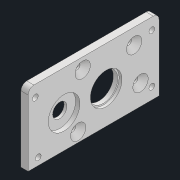
# Autodesk Inventor part: One Motor Plate
Saved by Autodesk Inventor 2022 (Build 260153000, 153)
## iProperties
Created: 2022-09-09
Part Number: One Motor Plate
Material: Generic
Document SubType Name: Modeling
Designer: robpl
Density: 1 g/cm^3
Appearance: Default
Author: robpl
Autodesk Inventor part; units mm, degrees
ref_plane "YZ Plane" through (0, 0, 0) normal (1, 0, 0) x (0, 1, 0)
ref_plane "XZ Plane" through (0, 0, 0) normal (0, 1, 0) x (-1, 0, 0)
ref_plane "XY Plane" through (0, 0, 0) normal (0, 0, 1) x (1, 0, 0)
sketch "Sketch1" plane through (0, 0, 0) normal (1, 0, 0) x (0, 1, 0)
  line L0 (0, 0) -> (50, 0)
  line L1 (50, 0) -> (50, -91)
  line L2 (50, -91) -> (0, -91)
  line L3 (0, -91) -> (0, 0)
  dimension "d0" = 50
  dimension "d1" = 91
  constraints: 8 end point, 2 parallel, 1 horizontal, 1 perpendicular
  measures "d0" distance of L1.end L2.end
  measures "d1" distance of L0.end L1.end
extrude "Extrusion1" add sketch "Sketch1" along normal blind 5
sketch "Sketch2" plane through (5, 0, 0) normal (1, 0, 0) x (0, 0, -1)
  line L0 (0, 0) -> (91, 0) projected
  line L1 (0, 50) -> (0, 0) projected
  point P0 (25, 22.8)
  dimension "d4" = 22.8
  dimension "d5" = 25
  measures "d4" distance from line of point (25, 22.8) L0
  measures "d5" distance from line of L1 point (25, 22.8)
hole "Hole1" at (5, 22.8, -25) direction (-1, 0, 0) diameter 10 end through all counterbore diameter 22 counterbore depth 3
sketch "Sketch3" plane through (5, 0, 0) normal (1, 0, 0) x (0, 0, -1)
  circle A0 centre (25, 22.8) radius 11 projected
  line L0 (91, 0) -> (91, 50) projected
  line L1 (91, 50) -> (0, 50) projected
  line L2 (0, 50) -> (0, 0) projected
  line L3 (0, 0) -> (91, 0) projected
  circle A1 centre (25, 22.8) radius 5 projected
  line L4 (25, 22.8) -> (54.26, 22.8)
  dimension "d13" = 29.26
  dimension "d14" = 0
  constraints: 2 end point, 1 coincident
  measures "d13" distance of L4.start L4.end
  measures "d14" angle of L3 L4
hole "Hole2" at (5, 22.8, -54.26) direction (-1, 0, 0) diameter 20 end through all counterbore diameter 22 counterbore depth 2
sketch "Sketch4" plane through (5, 0, 0) normal (1, 0, 0) x (0, 0, -1)
  circle A0 centre (54.26, 22.8) radius 11 projected
  line L0 (54.26, 22.8) -> (73.7175, 39.1268)
  line L1 (0, 0) -> (91, 0) projected
  point P0 (49.8493, 47.8141)
  point P1 (30.3918, 31.4873)
  point P2 (34.8025, 6.4732)
  point P3 (58.6707, -2.2141)
  point P4 (78.1282, 14.1127)
  dimension "d22" = 25.4
  dimension "d23" = 40
  dimension "d33" = 360
  constraints: 2 end point, 1 coincident, 7 other
  measures "d22" distance of L0.start L0.end
  measures "d23" angle of L1 L0
hole "Falcon Bolt Holes" at (5, 39.1268, -73.7175) at (5, 6.4732, -34.8025) at (5, 14.1127, -78.1282) direction (-1, 0, 0) diameter 4 end through all countersink diameter 10.668 countersink angle 82
fillet "Fillet1" radius 4 2 edges at (2.5, 50, 0) (2.5, 50, -91)
sketch "Sketch8" plane through (5, 0, 0) normal (1, 0, 0) x (0, 0, -1)
  line L0 (87, 50) -> (4, 50) projected
  line L1 (91, 0) -> (91, 46) projected
  line L2 (0, 0) -> (91, 0) projected
  line L3 (0, 46) -> (0, 0) projected
  circle A0 centre (5, 42) radius 4.5
  circle A1 centre (5, 42) radius 2
  circle A2 centre (7, 5) radius 4.5
  circle A3 centre (7, 5) radius 2
  circle A4 centre (86, 42) radius 4.5
  circle A5 centre (86, 42) radius 2
  circle A6 centre (86, 8) radius 4.5
  circle A7 centre (86, 8) radius 2
  dimension "d55" = 8
  dimension "d57" = 5
  dimension "d58" = 8
  dimension "d59" = 7
  dimension "d60" = 5
  dimension "d61" = 5
  dimension "d62" = 8
  dimension "d63" = 9
  dimension "d64" = 4
  dimension "d65" = 9
  dimension "d66" = 4
  dimension "d67" = 9
  dimension "d68" = 4
  dimension "d69" = 9
  dimension "d70" = 4
  dimension "d71" = 5
  constraints: 8 centre point, 8 coincident
  measures "d55" distance from line of L0 point (86, 42)
  measures "d57" distance from line of L1 point (86, 42)
  measures "d58" distance from line of L2 point (86, 8)
  measures "d59" distance from line of L3 point (7, 5)
  measures "d60" distance from line of L2 point (7, 5)
  measures "d61" distance from line of L3 point (5, 42)
  measures "d62" distance from line of L0 point (5, 42)
  measures "d63" diameter of A0
  measures "d64" diameter of A1
  measures "d65" diameter of A2
  measures "d66" diameter of A3
  measures "d67" diameter of A4
  measures "d68" diameter of A5
  measures "d69" diameter of A6
  measures "d70" diameter of A7
  measures "d71" distance from line of L1 A6.centre
hole "Hole5" at (5, 42, -5) at (5, 42, -86) at (5, 8, -86) at (5, 5, -7) direction (-1, 0, 0) diameter 4 end through all
sketch "Sketch10" plane through (5, 0, 0) normal (1, 0, 0) x (0, 0, -1)
  circle A0 centre (54.26, 22.8) radius 11 projected
  line L0 (37.9332, 42.2575) -> (73.7175, 39.1268)
  line L1 (73.7175, 39.1268) -> (70.5868, 3.3425)
  line L2 (70.5868, 3.3425) -> (34.8025, 6.4732)
  line L3 (34.8025, 6.4732) -> (37.9332, 42.2575)
  line L4 (54.26, 22.8) -> (37.9332, 42.2575)
  line L5 (0, 46) -> (0, 0) projected
  line L6 (91, 0) -> (91, 46) projected
  line L7 (0, 0) -> (91, 0)
  circle A1 centre (34.8025, 6.4732) radius 2 projected
  dimension "d81" = 25.4
  dimension "d82" = 5
  constraints: 12 end point, 4 coincident, 1 horizontal, 9 other
  measures "d81" distance of L4.start L0.start
  measures "d82" angle of L2 L7
hole "Neo Bolt Holes" at (5, 42.2575, -37.9332) at (5, 39.1268, -73.7175) at (5, 6.4732, -34.8025) direction (-1, 0, 0) diameter 4 end through all countersink diameter 10.668 countersink angle 82
body "Solid1"
